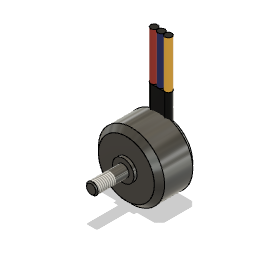
_2206 motor.c132166b-7eeb-4be8-b820-1d2212d54bd5 (Autodesk Fusion 360 design; units mm, degrees)
Autodesk Fusion 360 part; units mm, degrees
sketch "Sketch1" plane through (0, 0, 0) normal (0, 0, 1) x (1, 0, 0)
  circle A0 centre (0, 0) radius 13.9
  circle A1 centre (0, 0) radius 2.5
  circle A2 centre (0, 0) radius 4.5
  circle A3 centre (0, 0) radius 11.75
  line L0 (0, 0) -> (0, 8)
  line L1 (0, 0) -> (0, -8)
  line L2 (0, 0) -> (-9.5, 0)
  line L3 (0, 0) -> (9.5, 0)
  line L4 (-4.5, -10.8541) -> (-4.5, -22.9)
  line L5 (4.5, -10.8541) -> (4.5, -22.9)
  line L6 (4.5, -22.9) -> (-4.5, -22.9)
  dimension "d1" = 27.8
  dimension "d2" = 5
  dimension "d3" = 9
  dimension "d4" = 23.5
  dimension "d17" = 8
  dimension "d18" = 8
  dimension "d19" = 9.5
  dimension "d20" = 9.5
  constraint coincident A0.centre A1.centre
  constraint concentric A0 A1
  constraint concentric A0 A2
  constraint concentric A2 A3
  constraint vertical L0
  constraint parallel L0 L1
  constraint perpendicular L0 L2
  constraint parallel L2 L3
  constraint perpendicular L4 L6
  constraint coincident A3 L5.start
  constraint coincident A3 L4.start
  measures "d1" diameter of A0
  measures "d2" diameter of A1
  measures "d3" diameter of A2
  measures "d4" diameter of A3
  measures "d17" distance of A0.centre L0.end
  measures "d18" distance of A0.centre L1.end
  measures "d19" distance of A0.centre L2.end
  measures "d20" distance of A0.centre L3.end
extrude "Extrude5" add sketch "Sketch1" along normal blind 3 contours A0 A3 L4 L5 | A0 L4 L5 L6 picked at (0, -13.1632) makes body 1
extrude "Extrude1" add sketch "Sketch1" along normal blind 16.2 separate body contours A3 makes body 2
extrude "Extrude2" add sketch "Sketch1" along normal blind 17.5 contours A1 A2 L1 L3 | A1 A2 L0 L3 | A1 A2 L0 L2 | A1 A2 L1 L2 bodies 2
extrude "Extrude3" add sketch "Sketch1" along normal blind 31 contours A1 L0 L3 | A1 L1 L3 | A1 L0 L2 | A1 L1 L2 bodies 2
extrude "Extrude4" add sketch "Sketch1" along normal blind 14 contours A0 A3 L4 L5 | A0 A3 L4 L5 bodies 2
chamfer "Chamfer1" distance 2.15 angle 45 1 edges at (-12.9594, -5.0265, 0) on bodies 2
chamfer "Chamfer2" distance 2.15 angle 45 1 edges at (-10.9548, -4.249, 14) on bodies 2
thread "Thread1" "ISO Metric profile 5.0 M5x0.8 6g" major diameter 4.901 minor diameter 3.9895 pitch 0.8 angle 60 resizes the face on face at (2.4876, -0.2489, 22) from (0, 0, 23) to (0, 0, 31) on bodies 2
hole "Hole1" at (-9.5, 0, 0) direction (0, 0, 1) diameter 2.529 depth 4 tip angle 118 bodies 2
thread "Thread2" "ISO Metric profile 3.0 M3x0.5 6H"
hole "Hole2" at (0, -8, 0) direction (0, 0, 1) diameter 2.529 depth 4 tip angle 118 bodies 2
thread "Thread3" "ISO Metric profile 3.0 M3x0.5 6H"
hole "Hole3" at (0, 8, 0) direction (0, 0, 1) diameter 2.529 depth 4 tip angle 118 bodies 2
thread "Thread4" "ISO Metric profile 3.0 M3x0.5 6H"
hole "Hole4" at (9.5, 0, 0) direction (0, 0, 1) diameter 2.529 depth 4 tip angle 118 bodies 2
thread "Thread5" "ISO Metric profile 3.0 M3x0.5 6H"
chamfer "Chamfer3" distance 0.5 angle 45 1 edges at (-2.2847, -0.8861, 31) on bodies 2
fillet "Fillet1" radius 1.5 4 edges at (-4.5, -16.8771, 3) (-4.5, -16.8771, 0) (4.5, -16.8771, 3) (4.5, -16.8771, 0) on bodies 1
sketch "Sketch2" plane through (0, -22.9, 0) normal (0, -1, 0) x (1, 0, 0)
  arc A0 (3, 0) -> (3, 3) centre (3, 1.5) ccw
  line L0 (3, 3) -> (-3, 3)
  arc A1 (-3, 3) -> (-3, 0) centre (-3, 1.5) ccw
  line L1 (-3, 0) -> (3, 0)
  circle A2 centre (-3, 1.5) radius 1.5
  circle A3 centre (3, 1.5) radius 1.5
  circle A4 centre (-0.0373, 1.5) radius 1.45
  circle A5 centre (3, 1.5) radius 1.45
  circle A6 centre (-3, 1.5) radius 1.45
  dimension "d40" = 2.9
  dimension "d41" = 2.9
  dimension "d42" = 2.9
  constraint concentric A1 A2
  constraint concentric A0 A3
  constraint concentric A0 A5
  constraint concentric A1 A6
  measures "d40" diameter of A4
  measures "d41" diameter of A5
  measures "d42" diameter of A6
extrude "Extrude6" add sketch "Sketch2" along normal blind 20 contours A4 | A5 | A6 bodies 1
move_body "Move1" bodies 1 2 to x (-1, 0, 0) y (0, -1, 0) z (0, 0, 1) at (0, 0, 0)
